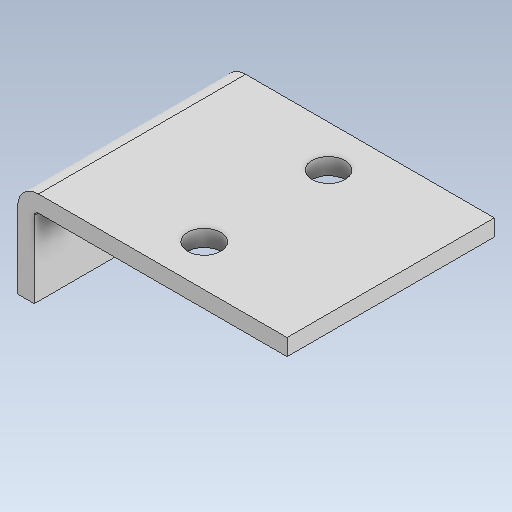
# Autodesk Inventor part: leche
Saved by Autodesk Inventor 2020 (Build 240168000, 168)
## iProperties
Created: 2020-10-05
Part Number: leche
Material: Genérico
Document SubType Name: Modeling
Designer: Pipi
Density: 1 g/cm^3
Appearance: Valor por defecto
Author: Pipi
Autodesk Inventor part; units mm, degrees
note: some values were not read from the file. Chosen so that the rebuilt part matches the saved one: bend side of "Pieza de plegado1".
ref_plane "YZ Plane" through (0, 0, 0) normal (1, 0, 0) x (0, 1, 0)
ref_plane "XZ Plane" through (0, 0, 0) normal (0, 1, 0) x (-1, 0, 0)
ref_plane "XY Plane" through (0, 0, 0) normal (0, 0, 1) x (1, 0, 0)
sketch "Boceto1" plane through (0, 0, 0) normal (0, 1, 0) x (-1, 0, 0)
  line L0 (7.2949, 12.862) -> (7.2949, -12.138)
  line L1 (7.2949, -12.138) -> (-32.7051, -12.138)
  line L2 (-32.7051, -12.138) -> (-32.7051, 12.862)
  line L3 (-32.7051, 12.862) -> (7.2949, 12.862)
  line L4 (-2.7051, -12.138) -> (-2.7051, 12.862)
  circle A0 centre (-17.7051, -7.138) radius 2
  circle A1 centre (-17.7051, 7.862) radius 2
  line L5 (7.2949, -12.138) -> (2.2949, -12.138)
  circle A2 centre (2.2949, -7.138) radius 2
  point P0 (0, 0)
  dimension "d0" = 25
  dimension "d1" = 40
  dimension "d11" = 4
  dimension "d12" = 4
  dimension "d13" = 5
  dimension "d14" = 5
  dimension "d15" = 15
  dimension "d16" = 15
  dimension "d18" = 4
  dimension "d19" = 5
  dimension "d20" = 5
  constraints: 12 end point, 4 perpendicular, 3 centre point, 3 point on line, 1 vertical
  measures "d0" distance of L0.start L0.end
  measures "d1" distance of L0.end L1.end
  measures "d11" diameter of A0
  measures "d12" diameter of A1
  measures "d13" distance from line of L1 A0.centre
  measures "d14" distance from line of L3 A1.centre
  measures "d15" distance from line of L2 A0.centre
  measures "d16" distance from line of L2 A1.centre
  measures "d18" diameter of A2
  measures "d19" distance from line of L0 A2.centre
  measures "d20" distance from line of L1 A2.centre
extrude "Extrusión2" add sketch "Boceto1" along normal blind 2 contours L4 L1 L2 L3
extrude "Extrusión3" add sketch "Boceto1" along normal blind 2 contours L0 L1 L4 L3
bend part "Pieza de plegado1" radius 0.5 angle 90 line through (2.7051, 0, -12.138) along (0, 0, 1) centre toward (0, -1, 0) moving side (-1, 0, 0) both sides no
